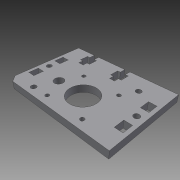
# Autodesk Inventor part: z_motor_mount_v2
Saved by Autodesk Inventor 2014 (Build 180170000, 170)
## iProperties
Created: 2013-12-06
Part Number: z_motor_mount_v2
Material: Generic
Document SubType Name: Modeling
Designer: buben
Density: 1 g/cm^3
Appearance: Default
Author: buben
Autodesk Inventor part; units mm, degrees
ref_plane "YZ Plane" through (0, 0, 0) normal (1, 0, 0) x (0, 1, 0)
ref_plane "XZ Plane" through (0, 0, 0) normal (0, 1, 0) x (-1, 0, 0)
ref_plane "XY Plane" through (0, 0, 0) normal (0, 0, 1) x (1, 0, 0)
sketch "Sketch1" plane through (0, 0, 0) normal (0, 0, 1) x (1, 0, 0)
  line L0 (5, 0) -> (90, 0)
  line L1 (90, 0) -> (90, 64)
  line L2 (90, 64) -> (0, 64)
  line L3 (0, 64) -> (0, 5)
  line L4 (0, 5) -> (5, 0)
  line L5 (33.5, 37.5) -> (64.5, 37.5) construction
  line L6 (64.5, 37.5) -> (64.5, 6.5) construction
  line L7 (64.5, 6.5) -> (33.5, 6.5) construction
  line L8 (33.5, 6.5) -> (33.5, 37.5) construction
  line L9 (27.62, 43.38) -> (70.38, 43.38) construction
  line L10 (70.38, 43.38) -> (70.38, 0.62) construction
  line L11 (70.38, 0.62) -> (27.62, 0.62) construction
  line L12 (27.62, 0.62) -> (27.62, 43.38) construction
  circle A0 centre (33.5, 6.5) radius 1.6
  circle A1 centre (64.5, 6.5) radius 1.6
  circle A2 centre (64.5, 37.5) radius 1.6
  circle A3 centre (33.5, 37.5) radius 1.6
  circle A4 centre (49, 22) radius 11.5
  circle A5 centre (26, 22) radius 4
  point P0 (0, 0)
  point P1 (49, 37.5)
  point P2 (64.5, 22)
  point P3 (70.38, 22)
  point P4 (49, 43.38)
  dimension "d0" = 45
  dimension "d1" = 31
  dimension "d2" = 42.76
  dimension "d3" = 3.2
  dimension "d4" = 23
  dimension "d5" = 8
  dimension "d6" = 23
  dimension "d7" = 41
  dimension "d8" = 90
  dimension "d9" = 42
  dimension "d10" = 5
  dimension "d11" = 22
  constraints: 26 end point, 6 centre point, 6 parallel, 5 perpendicular, 4 coincident, 4 horizontal alignment, 4 midpoint, 3 equal radius, 3 horizontal, 3 vertical alignment
  measures "d0" angle of L0 L4
  measures "d1" distance of L6.end L7.end
  measures "d2" distance of L10.end L11.end
  measures "d3" diameter of A0
  measures "d4" diameter of A4
  measures "d5" diameter of A5
  measures "d6" distance of A4.centre A5.centre
  measures "d7" distance from line of L1 A4.centre
  measures "d8" distance of L1.end L2.end
  measures "d9" distance from line of L2 A5.centre
  measures "d10" horizontal distance of L0.start L3.end
  measures "d11" distance from line of L0 A5.centre
extrude "Extrusion1" add sketch "Sketch1" along normal blind 6
sketch "Sketch3" plane through (0, 0, 6) normal (0, 0, 1) x (1, 0, 0)
  circle A0 centre (26, 22) radius 4 projected
  circle A1 centre (64.5, 37.5) radius 1.6 projected
  line L0 (5, 0) -> (90, 0) projected
  circle A2 centre (20, 6) radius 2.25
  circle A3 centre (70.5, 49.5) radius 2.25
  point P0 (0, 0)
  dimension "d29" = 4.5
  dimension "d30" = 6
  dimension "d31" = 6
  dimension "d32" = 12
  dimension "d33" = 6
  constraints: 2 centre point, 1 equal radius
  measures "d29" diameter of A3
  measures "d30" horizontal distance of A0.centre A2.centre
  measures "d31" distance from line of L0 A2.centre
  measures "d32" vertical distance of A1.centre A3.centre
  measures "d33" horizontal distance of A3.centre A1.centre
extrude "Extrusion3" cut sketch "Sketch3" against normal through all contours A2 | A3
sketch "Sketch4" plane through (0, 0, 6) normal (0, 0, 1) x (1, 0, 0)
  line L0 (90, 0) -> (90, 64) projected
  line L1 (0, 64) -> (0, 5) projected
  line L2 (5, 0) -> (90, 0) projected
  line L3 (3, 22) -> (9, 22)
  line L4 (9, 22) -> (9, 14)
  line L5 (9, 14) -> (3, 14)
  line L6 (3, 14) -> (3, 22)
  line L7 (3, 45) -> (9, 45)
  line L8 (9, 45) -> (9, 37)
  line L9 (9, 37) -> (3, 37)
  line L10 (3, 37) -> (3, 45)
  line L11 (81, 45) -> (87, 45)
  line L12 (87, 45) -> (87, 37)
  line L13 (87, 37) -> (81, 37)
  line L14 (81, 37) -> (81, 45)
  line L15 (81, 22) -> (87, 22)
  line L16 (87, 22) -> (87, 14)
  line L17 (87, 14) -> (81, 14)
  line L18 (81, 14) -> (81, 22)
  line L19 (3, 37) -> (9, 22) construction
  line L20 (3, 22) -> (9, 37) construction
  line L21 (81, 37) -> (87, 22) construction
  line L22 (81, 22) -> (87, 37) construction
  circle A0 centre (6, 29.5) radius 2.25
  circle A1 centre (84, 29.5) radius 2.25
  point P0 (0, 0)
  dimension "d36" = 6
  dimension "d37" = 8
  dimension "d38" = 8
  dimension "d39" = 6
  dimension "d40" = 15
  dimension "d41" = 3
  dimension "d42" = 3
  dimension "d43" = 14
  dimension "d44" = 4.5
  constraints: 40 end point, 8 collinear, 8 parallel, 4 horizontal, 4 perpendicular, 2 centre point, 2 midpoint, 1 equal radius
  measures "d36" distance of L7.start L7.end
  measures "d37" distance of L9.end L7.start
  measures "d38" distance of L5.end L3.start
  measures "d39" distance of L11.start L11.end
  measures "d40" distance between parallel lines of L3 L9
  measures "d41" distance between parallel lines of L1 L10
  measures "d42" distance between parallel lines of L0 L12
  measures "d43" distance between parallel lines of L2 L5
  measures "d44" diameter of A0
extrude "Extrusion4" cut sketch "Sketch4" against normal through all
sketch "Sketch5" plane through (0, 0, 6) normal (0, 0, 1) x (1, 0, 0)
  line L0 (90, 64) -> (0, 64) projected
  line L1 (0, 64) -> (0, 5) projected
  line L2 (17.75, 64) -> (22.25, 64)
  line L3 (22.25, 47.7) -> (17.75, 47.7)
  line L4 (24.75, 59) -> (24.75, 51.7)
  line L5 (15.25, 51.7) -> (15.25, 59)
  line L6 (17.75, 47.7) -> (17.75, 51.7)
  line L7 (17.75, 59) -> (17.75, 64)
  line L8 (22.25, 64) -> (22.25, 59)
  line L9 (22.25, 51.7) -> (22.25, 47.7)
  line L10 (15.25, 59) -> (17.75, 59)
  line L11 (22.25, 59) -> (24.75, 59)
  line L12 (24.75, 51.7) -> (22.25, 51.7)
  line L13 (17.75, 51.7) -> (15.25, 51.7)
  line L14 (47.75, 64) -> (52.25, 64)
  line L15 (52.25, 47.7) -> (47.75, 47.7)
  line L16 (54.75, 59) -> (54.75, 51.7)
  line L17 (45.25, 51.7) -> (45.25, 59)
  line L18 (47.75, 47.7) -> (47.75, 51.7)
  line L19 (47.75, 59) -> (47.75, 64)
  line L20 (52.25, 64) -> (52.25, 59)
  line L21 (52.25, 51.7) -> (52.25, 47.7)
  line L22 (45.25, 59) -> (47.75, 59)
  line L23 (52.25, 59) -> (54.75, 59)
  line L24 (54.75, 51.7) -> (52.25, 51.7)
  line L25 (47.75, 51.7) -> (45.25, 51.7)
  point P0 (0, 0)
  point P1 (20, 47.7)
  point P2 (50, 47.7)
  dimension "d47" = 4.5
  dimension "d48" = 2.5
  dimension "d49" = 2.5
  dimension "d50" = 5
  dimension "d51" = 7.3
  dimension "d52" = 4
  dimension "d53" = 4.5
  dimension "d54" = 2.5
  dimension "d55" = 2.5
  dimension "d56" = 5
  dimension "d57" = 7.3
  dimension "d58" = 4
  dimension "d59" = 20
  dimension "d60" = 30
  constraints: 48 end point, 20 parallel, 10 collinear, 8 perpendicular, 6 horizontal, 2 midpoint
  measures "d47" distance of L3.start L3.end
  measures "d48" distance of L6.end L5.start
  measures "d49" distance of L4.end L9.start
  measures "d50" distance of L2.end L8.end
  measures "d51" distance of L4.start L4.end
  measures "d52" distance of L9.start L3.start
  measures "d53" distance of L21.end L15.end
  measures "d54" distance of L18.end L25.end
  measures "d55" distance of L24.start L24.end
  measures "d56" distance of L14.end L23.start
  measures "d57" distance of L23.end L24.start
  measures "d58" distance of L24.end L21.end
  measures "d59" distance from line of L1 point (20, 47.7)
  measures "d60" distance of point (20, 47.7) point (50, 47.7)
extrude "Extrusion5" cut sketch "Sketch5" against normal through all
body "Solid1"
